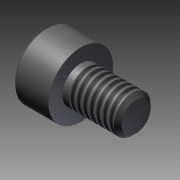
# Autodesk Inventor part: SCB4-6_1
Saved by Autodesk Inventor 2011 SP1 (Build 150282100, 282)
## iProperties
Created: 2015-02-01
Part Number: SCB4-6_1
Catalog Web Link: www.cadenas.de
Description: SCB_1-Hexagon Socket Head Cap Screws - Stainless Steel
Vendor: MISUMI
Document SubType Name: Modeling
Designer: PARTuser1
Manufacturer: MISUMI
Mass: 0.210032 g
Surface Area: 2.52603 cm^2
Volume: 0.210032 cm^3
Density: 1 g/cm^3
Category: PARTsolutions
Company: MISUMI
Title: SCB4-6_1
Author: Cadenas PARTsolutions
Comments: Hexagon Socket Head Cap Screws - Stainless Steel
PSOL_IDENT_0: {\\10.0.0.236\data_v8\23d-libs\misumi\metric\27_screws_nuts\scb.prj},158 {VTYP=3D},{NB=SCB4-6_1},{LI
PSOL_IDENT_1: NA=SCB4-6_1},{NN=SCB_1},{DATE=17.11.2014 07:44:00},{GEOMDATE=13.05.2010 00:00:00},{VERSION=},{LINEID=
PSOL_IDENT_2: 50},{LINESUBID=-1},{WBVAR=L}  {NB=SCB4-6_1},{LINA=SCB4-6_1},{KT=DUMMY},{PN=SCB4-6},{MAT=SUSXM7(30430
PSOL_IDENT_3: Stainless Steel)},{SC=A2-70},{M=4},{L=6},{LL=Full Thread},{L1=20},{TYPE=SCB},{M1=4.0},{M2=4.0},{L0=
PSOL_IDENT_4: 6,8,10,12,15,20,25,30,35,40,45},{MP=4x0.7},{P=0.7},{A=7.0},{E=4.0},{B=3.0},{V=0.40}
SUPPLIER: MISUMI
ARTICLENO: SCB4-6_1
BOMINFO: SCB4-6_1
CREATOR: CADENAS GmbH
Autodesk Inventor part; units mm, degrees
sketch "Sketch_1" plane through (0, 0, 0) normal (0, 0, 1) x (1, 0, 0)
  line L0 (6, 0) -> (-4, 0)
  line L1 (-4, 0) -> (-4, 3.1)
  line L2 (-4, 3.1) -> (-3.6, 3.5)
  line L3 (-3.6, 3.5) -> (0, 3.5)
  line L4 (0, 3.5) -> (0, 2)
  line L5 (0, 2) -> (5.5705, 2)
  line L6 (5.5705, 2) -> (6, 1.5705)
  line L7 (6, 1.5705) -> (6, 0)
  line L8 (6, 0) -> (-4, 0)
  constraints: 18 end point
revolve "Revolution1" add sketch "Sketch_1" angle 360 about axis through (6, 0, 0) along (1, 0, 0)
thread "Thread1" size "M4x0.7" class "6g" standard "ISO Metric profile" length 5.3 offset 0.7
sketch "Sketch_4" plane through (0, 0, 0) normal (0, 0, 1) x (1, 0, 0)
  line L0 (-1.5981, 0) -> (-4, 0)
  line L1 (-4, 0) -> (-4, 1.5)
  line L2 (-4, 1.5) -> (-2, 1.5)
  line L3 (-2, 1.5) -> (-1.5981, 0)
  line L4 (-1.5981, 0) -> (-4, 0)
  constraints: 10 end point
revolve "Revolution2" cut sketch "Sketch_4" angle 360 about axis through (-1.5981, 0, 0) along (1, 0, 0)
sketch "Sketch_3" plane through (-4, 0, 0) normal (1, 0, 0) x (0, 0, -1)
  line L0 (-1.5, 0.866) -> (-1.5, -0.866)
  line L1 (-1.5, -0.866) -> (0, -1.7321)
  line L2 (0, -1.7321) -> (1.5, -0.866)
  line L3 (1.5, -0.866) -> (1.5, 0.866)
  line L4 (1.5, 0.866) -> (0, 1.7321)
  line L5 (0, 1.7321) -> (-1.5, 0.866)
  constraints: 12 end point
extrude "Extrusion1" cut sketch "Sketch_3" along normal blind 2
ref_plane "nut_XY" through (6, 0, 0) normal (1, 0, 0) x (0, 0, -1)
ref_plane "nut_YZ" through (6, 0, 0) normal (0, 0, -1) x (0, 1, 0)
ref_plane "nut_ZX" through (6, 0, 0) normal (0, 1, 0) x (1, 0, 0)
ref_plane "bolt_XY" through (0, 0, 0) normal (1, 0, 0) x (0, 0, -1)
ref_plane "bolt_YZ" through (0, 0, 0) normal (0, 0, -1) x (0, 1, 0)
ref_plane "bolt_ZX" through (0, 0, 0) normal (0, 1, 0) x (1, 0, 0)
body "Solid1"
